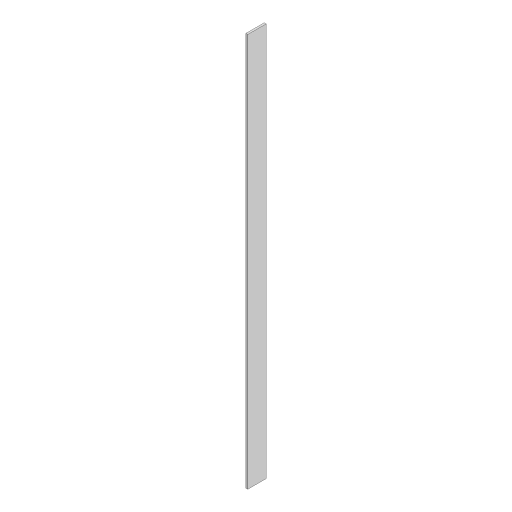
# Autodesk Inventor part: PLETINA PARA CAJA
Saved by Autodesk Inventor 2024 (Build 280153000, 153)
## iProperties
Created: 2024-07-05
Part Number: PLETINA PARA CAJA
Material: Generic
Document SubType Name: Modeling
Designer: Jhuliams
Density: 1 g/cm^3
Appearance: Default
Author: Jhuliams
Autodesk Inventor part; units mm, degrees
ref_plane "YZ Plane" through (0, 0, 0) normal (1, 0, 0) x (0, 1, 0)
ref_plane "XZ Plane" through (0, 0, 0) normal (0, 1, 0) x (-1, 0, 0)
ref_plane "XY Plane" through (0, 0, 0) normal (0, 0, 1) x (1, 0, 0)
sketch "Sketch1" plane through (0, 0, 0) normal (0, 1, 0) x (-1, 0, 0)
  line L0 (1.375, 12.7) -> (-1.375, 12.7)
  line L1 (-1.375, 12.7) -> (-1.375, -12.7)
  line L2 (-1.375, -12.7) -> (1.375, -12.7)
  line L3 (1.375, -12.7) -> (1.375, 12.7)
  line L4 (1.375, 12.7) -> (-1.375, -12.7) construction
  line L5 (-1.375, 12.7) -> (1.375, -12.7) construction
  point P0 (0, 0)
  dimension "d0" = 2.75
  dimension "d1" = 25.4
  constraints: 12 end point, 2 midpoint, 2 parallel, 1 horizontal, 1 perpendicular
  measures "d0" distance of L2.end L1.end
  measures "d1" distance of L1.end L0.end
extrude "Extrusion1" add sketch "Sketch1" along normal blind 545
body "Solid1"
